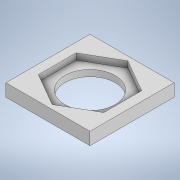
# Autodesk Inventor part: ScrewTest
Saved by Autodesk Inventor 2022 (Build 260153000, 153)
## iProperties
Created: 2022-04-20
Part Number: ScrewTest
Material: Generic
Document SubType Name: Modeling
Designer: Bruger
Density: 1 g/cm^3
Appearance: Default
Author: Bruger
Autodesk Inventor part; units mm, degrees
ref_plane "YZ Plane" through (0, 0, 0) normal (1, 0, 0) x (0, 1, 0)
ref_plane "XZ Plane" through (0, 0, 0) normal (0, 1, 0) x (-1, 0, 0)
ref_plane "XY Plane" through (0, 0, 0) normal (0, 0, 1) x (1, 0, 0)
sketch "Sketch1" plane through (0, 0, 0) normal (0, 1, 0) x (-1, 0, 0)
  line L0 (-10, 10) -> (10, 10)
  line L1 (10, 10) -> (10, -10)
  line L2 (10, -10) -> (-10, -10)
  line L3 (-10, -10) -> (-10, 10)
  line L4 (-10, 10) -> (10, -10) construction
  line L5 (10, 10) -> (-10, -10) construction
  circle A0 centre (0, 0) radius 6
  line L6 (0, 0) -> (0, -9)
  line L7 (0, 0) -> (9, 0)
  line L8 (0, 0) -> (7.7942, -4.5)
  line L9 (0, 0) -> (-7.7942, -4.5)
  line L10 (0, 0) -> (9, 0) construction
  line L11 (0, 0) -> (-7.7942, -4.5)
  line L12 (0, 0) -> (9, 0) construction
  line L13 (0, 0) -> (0, 9)
  line L14 (0, 0) -> (7.7942, 4.5)
  line L15 (0, 0) -> (9, 0) construction
  line L16 (0, 0) -> (-7.7942, 4.5)
  line L17 (0, 0) -> (9, 0) construction
  line L18 (0, -9) -> (-7.7942, -4.5)
  line L19 (-7.7942, -4.5) -> (-7.7942, 4.5)
  line L20 (-7.7942, 4.5) -> (0, 9)
  line L21 (0, 9) -> (7.7942, 4.5)
  line L22 (7.7942, 4.5) -> (7.7942, -4.5)
  line L23 (7.7942, -4.5) -> (0, -9)
  dimension "d0" = 20
  dimension "d1" = 20
  dimension "d2" = 12
  dimension "d11" = 9
  dimension "d14" = 9
  dimension "d15" = 9
  dimension "d16" = 150
  dimension "d17" = 9
  dimension "d18" = 210
  dimension "d19" = 9
  dimension "d20" = 9
  dimension "d21" = 30
  dimension "d22" = 9
  dimension "d23" = 150
  constraints: 48 end point, 6 horizontal, 5 parallel, 4 equal length, 2 midpoint, 2 perpendicular, 1 centre point, 1 coincident, 1 vertical
  measures "d0" distance of L1.end L2.end
  measures "d1" distance of L0.end L1.end
  measures "d2" diameter of A0
  measures "d11" distance of L6.start L6.end
  measures "d14" distance of L6.start L8.end
  measures "d15" distance of L6.start L9.end
  measures "d16" angle of L9 L10
  measures "d17" distance of L6.start L9.end
  measures "d19" distance of L6.start L13.end
  measures "d20" distance of L6.start L14.end
  measures "d21" angle of L15 L14
  measures "d22" distance of L6.start L16.end
  measures "d23" angle of L17 L16
extrude "Extrusion1" add sketch "Sketch1" along normal blind 3 contours L0 L1 L2 L3 | L7 L14 A0 | L7 L22 L8 A0 | A0 L8 L7 | A0 L14 L22 L7 | L14 L13 A0 | A0 L13 L21 L14 | L8 L23 L6 A0 | A0 L6 L8 | L6 A0 L9 | L16 A0 L13 | L9 A0 L16 | A0 L16 L20 L13 | L6 L18 L9 A0 | L9 L19 L16 A0
extrude "Extrusion4" cut sketch "Sketch1" along normal blind 9 contours L7 L14 A0 | L7 L22 L8 A0 | A0 L8 L7 | A0 L14 L22 L7 | L14 L13 A0 | A0 L13 L21 L14 | L8 L23 L6 A0 | A0 L6 L8 | L6 A0 L9 | L16 A0 L13 | L9 A0 L16 | A0 L16 L20 L13 | L6 L18 L9 A0 | L9 L19 L16 A0
extrude "Extrusion5" add sketch "Sketch1" along normal blind 1.5 contours L7 L22 L8 A0 | A0 L14 L22 L7 | A0 L13 L21 L14 | L8 L23 L6 A0 | A0 L16 L20 L13 | L6 L18 L9 A0 | L9 L19 L16 A0
body "Solid1"
